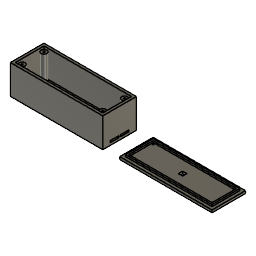
CajaSensorHumedad_v1 (Autodesk Fusion 360 design; units mm, degrees)
part number: 2026-06-22-22-06-37-882
Autodesk Fusion 360 part; units mm, degrees
sketch "Boceto1" plane through (0, 0, 0) normal (0, 0, 1) x (1, 0, 0)
sketch "Boceto2" plane through (0, 0, 0) normal (0, 0, 1) x (1, 0, 0)
sketch "Boceto3" plane through (0, 0, 0) normal (0, 0, 1) x (1, 0, 0)
  line L0 (0, 0) -> (110, 0)
  line L1 (110, 0) -> (110, 40)
  line L2 (110, 40) -> (0, 40)
  line L3 (0, 40) -> (0, 0)
sketch "Boceto4" plane through (0, 0, 0) normal (0, 0, 1) x (1, 0, 0)
  line L0 (0, 0) -> (110, 0)
  line L1 (110, 0) -> (110, 3)
  line L2 (110, 3) -> (0, 3)
  line L3 (0, 3) -> (0, 0)
sketch "Boceto5" plane through (0, 0, 0) normal (0, 0, 1) x (1, 0, 0)
  line L0 (0, 37) -> (110, 37)
  line L1 (110, 37) -> (110, 40)
  line L2 (110, 40) -> (0, 40)
  line L3 (0, 40) -> (0, 37)
sketch "Boceto6" plane through (0, 0, 0) normal (0, 0, 1) x (1, 0, 0)
  line L0 (0, 0) -> (3, 0)
  line L1 (3, 0) -> (3, 13)
  line L2 (3, 13) -> (0, 13)
  line L3 (0, 13) -> (0, 0)
sketch "Boceto7" plane through (0, 0, 0) normal (0, 0, 1) x (1, 0, 0)
  line L0 (0, 27) -> (3, 27)
  line L1 (3, 27) -> (3, 40)
  line L2 (3, 40) -> (0, 40)
  line L3 (0, 40) -> (0, 27)
sketch "Boceto8" plane through (0, 0, 0) normal (0, 0, 1) x (1, 0, 0)
  line L0 (0, 13) -> (3, 13)
  line L1 (3, 13) -> (3, 27)
  line L2 (3, 27) -> (0, 27)
  line L3 (0, 27) -> (0, 13)
sketch "Boceto9" plane through (0, 0, 0) normal (0, 0, 1) x (1, 0, 0)
  line L0 (107, 0) -> (110, 0)
  line L1 (110, 0) -> (110, 9)
  line L2 (110, 9) -> (107, 9)
  line L3 (107, 9) -> (107, 0)
sketch "Boceto10" plane through (0, 0, 0) normal (0, 0, 1) x (1, 0, 0)
  line L0 (107, 19) -> (110, 19)
  line L1 (110, 19) -> (110, 21)
  line L2 (110, 21) -> (107, 21)
  line L3 (107, 21) -> (107, 19)
sketch "Boceto11" plane through (0, 0, 0) normal (0, 0, 1) x (1, 0, 0)
  line L0 (107, 31) -> (110, 31)
  line L1 (110, 31) -> (110, 40)
  line L2 (110, 40) -> (107, 40)
  line L3 (107, 40) -> (107, 31)
sketch "Boceto12" plane through (0, 0, 0) normal (0, 0, 1) x (1, 0, 0)
  line L0 (107, 9) -> (110, 9)
  line L1 (110, 9) -> (110, 31)
  line L2 (110, 31) -> (107, 31)
  line L3 (107, 31) -> (107, 9)
sketch "Boceto13" plane through (0, 0, 0) normal (0, 0, 1) x (1, 0, 0)
  circle A0 centre (7, 7) radius 3.5
sketch "Boceto14" plane through (0, 0, 0) normal (0, 0, 1) x (1, 0, 0)
  circle A0 centre (7, 7) radius 1.1
sketch "Boceto15" plane through (0, 0, 0) normal (0, 0, 1) x (1, 0, 0)
  circle A0 centre (103, 7) radius 3.5
sketch "Boceto16" plane through (0, 0, 0) normal (0, 0, 1) x (1, 0, 0)
  circle A0 centre (103, 7) radius 1.1
sketch "Boceto17" plane through (0, 0, 0) normal (0, 0, 1) x (1, 0, 0)
  circle A0 centre (7, 33) radius 3.5
sketch "Boceto18" plane through (0, 0, 0) normal (0, 0, 1) x (1, 0, 0)
  circle A0 centre (7, 33) radius 1.1
sketch "Boceto19" plane through (0, 0, 0) normal (0, 0, 1) x (1, 0, 0)
  circle A0 centre (103, 33) radius 3.5
sketch "Boceto20" plane through (0, 0, 0) normal (0, 0, 1) x (1, 0, 0)
  circle A0 centre (103, 33) radius 1.1
sketch "Boceto21" plane through (0, 0, 0) normal (0, 0, 1) x (1, 0, 0)
  circle A0 centre (35, 12) radius 2.5
sketch "Boceto22" plane through (0, 0, 0) normal (0, 0, 1) x (1, 0, 0)
  circle A0 centre (35, 12) radius 1.1
sketch "Boceto23" plane through (0, 0, 0) normal (0, 0, 1) x (1, 0, 0)
  circle A0 centre (75, 12) radius 2.5
sketch "Boceto24" plane through (0, 0, 0) normal (0, 0, 1) x (1, 0, 0)
  circle A0 centre (75, 12) radius 1.1
sketch "Boceto25" plane through (0, 0, 0) normal (0, 0, 1) x (1, 0, 0)
  circle A0 centre (35, 28) radius 2.5
sketch "Boceto26" plane through (0, 0, 0) normal (0, 0, 1) x (1, 0, 0)
  circle A0 centre (35, 28) radius 1.1
sketch "Boceto27" plane through (0, 0, 0) normal (0, 0, 1) x (1, 0, 0)
  circle A0 centre (75, 28) radius 2.5
sketch "Boceto28" plane through (0, 0, 0) normal (0, 0, 1) x (1, 0, 0)
  circle A0 centre (75, 28) radius 1.1
sketch "Boceto29" plane through (0, 0, 0) normal (0, 0, 1) x (1, 0, 0)
  circle A0 centre (95, 20) radius 3
sketch "Boceto30" plane through (0, 0, 0) normal (0, 0, 1) x (1, 0, 0)
  circle A0 centre (95, 20) radius 1.6
sketch "Boceto31" plane through (0, 0, 0) normal (0, 0, 1) x (1, 0, 0)
  circle A0 centre (53, 20) radius 2.5
sketch "Boceto32" plane through (0, 0, 0) normal (0, 0, 1) x (1, 0, 0)
  circle A0 centre (53, 20) radius 1.1
sketch "Boceto33" plane through (0, 0, 0) normal (0, 0, 1) x (1, 0, 0)
  circle A0 centre (57, 20) radius 2.5
sketch "Boceto34" plane through (0, 0, 0) normal (0, 0, 1) x (1, 0, 0)
  circle A0 centre (57, 20) radius 1.1
sketch "Boceto35" plane through (0, 0, 0) normal (0, 0, 1) x (1, 0, 0)
  line L0 (130, 0) -> (240, 0)
  line L1 (240, 0) -> (240, 40)
  line L2 (240, 40) -> (130, 40)
  line L3 (130, 40) -> (130, 0)
sketch "Boceto36" plane through (0, 0, 0) normal (0, 0, 1) x (1, 0, 0)
  line L0 (133.5, 3.5) -> (236.5, 3.5)
  line L1 (236.5, 3.5) -> (236.5, 5.5)
  line L2 (236.5, 5.5) -> (133.5, 5.5)
  line L3 (133.5, 5.5) -> (133.5, 3.5)
sketch "Boceto37" plane through (0, 0, 0) normal (0, 0, 1) x (1, 0, 0)
  line L0 (133.5, 34.5) -> (236.5, 34.5)
  line L1 (236.5, 34.5) -> (236.5, 36.5)
  line L2 (236.5, 36.5) -> (133.5, 36.5)
  line L3 (133.5, 36.5) -> (133.5, 34.5)
sketch "Boceto38" plane through (0, 0, 0) normal (0, 0, 1) x (1, 0, 0)
  line L0 (133.5, 3.5) -> (135.5, 3.5)
  line L1 (135.5, 3.5) -> (135.5, 36.5)
  line L2 (135.5, 36.5) -> (133.5, 36.5)
  line L3 (133.5, 36.5) -> (133.5, 3.5)
sketch "Boceto39" plane through (0, 0, 0) normal (0, 0, 1) x (1, 0, 0)
  line L0 (234.5, 3.5) -> (236.5, 3.5)
  line L1 (236.5, 3.5) -> (236.5, 36.5)
  line L2 (236.5, 36.5) -> (234.5, 36.5)
  line L3 (234.5, 36.5) -> (234.5, 3.5)
sketch "Boceto40" plane through (0, 0, 0) normal (0, 0, 1) x (1, 0, 0)
  line L0 (182.5, 17.5) -> (187.5, 17.5)
  line L1 (187.5, 17.5) -> (187.5, 22.5)
  line L2 (187.5, 22.5) -> (182.5, 22.5)
  line L3 (182.5, 22.5) -> (182.5, 17.5)
sketch "Boceto41" plane through (0, 0, 0) normal (0, 0, 1) x (1, 0, 0)
  circle A0 centre (137, 7) radius 1.1
sketch "Boceto42" plane through (0, 0, 0) normal (0, 0, 1) x (1, 0, 0)
  circle A0 centre (233, 7) radius 1.1
sketch "Boceto43" plane through (0, 0, 0) normal (0, 0, 1) x (1, 0, 0)
  circle A0 centre (137, 33) radius 1.1
sketch "Boceto44" plane through (0, 0, 0) normal (0, 0, 1) x (1, 0, 0)
  circle A0 centre (233, 33) radius 1.1
sketch "Boceto45" plane through (0, 0, 0) normal (0, 0, 1) x (1, 0, 0)
  line L0 (0, 0) -> (110, 0)
  line L1 (110, 0) -> (110, 40)
  line L2 (110, 40) -> (0, 40)
  line L3 (0, 40) -> (0, 0)
sketch "Boceto46" plane through (0, 0, 0) normal (0, 0, 1) x (1, 0, 0)
  line L0 (0, 0) -> (110, 0)
  line L1 (110, 0) -> (110, 3)
  line L2 (110, 3) -> (0, 3)
  line L3 (0, 3) -> (0, 0)
sketch "Boceto47" plane through (0, 0, 0) normal (0, 0, 1) x (1, 0, 0)
  line L0 (0, 37) -> (110, 37)
  line L1 (110, 37) -> (110, 40)
  line L2 (110, 40) -> (0, 40)
  line L3 (0, 40) -> (0, 37)
sketch "Boceto48" plane through (0, 0, 0) normal (0, 0, 1) x (1, 0, 0)
  line L0 (0, 0) -> (3, 0)
  line L1 (3, 0) -> (3, 13)
  line L2 (3, 13) -> (0, 13)
  line L3 (0, 13) -> (0, 0)
sketch "Boceto49" plane through (0, 0, 0) normal (0, 0, 1) x (1, 0, 0)
  line L0 (0, 27) -> (3, 27)
  line L1 (3, 27) -> (3, 40)
  line L2 (3, 40) -> (0, 40)
  line L3 (0, 40) -> (0, 27)
sketch "Boceto50" plane through (0, 0, 0) normal (0, 0, 1) x (1, 0, 0)
  line L0 (0, 13) -> (3, 13)
  line L1 (3, 13) -> (3, 27)
  line L2 (3, 27) -> (0, 27)
  line L3 (0, 27) -> (0, 13)
sketch "Boceto51" plane through (0, 0, 0) normal (0, 0, 1) x (1, 0, 0)
  line L0 (107, 0) -> (110, 0)
  line L1 (110, 0) -> (110, 9)
  line L2 (110, 9) -> (107, 9)
  line L3 (107, 9) -> (107, 0)
sketch "Boceto52" plane through (0, 0, 0) normal (0, 0, 1) x (1, 0, 0)
  line L0 (107, 19) -> (110, 19)
  line L1 (110, 19) -> (110, 21)
  line L2 (110, 21) -> (107, 21)
  line L3 (107, 21) -> (107, 19)
sketch "Boceto53" plane through (0, 0, 0) normal (0, 0, 1) x (1, 0, 0)
  line L0 (107, 31) -> (110, 31)
  line L1 (110, 31) -> (110, 40)
  line L2 (110, 40) -> (107, 40)
  line L3 (107, 40) -> (107, 31)
sketch "Boceto54" plane through (0, 0, 0) normal (0, 0, 1) x (1, 0, 0)
  line L0 (107, 9) -> (110, 9)
  line L1 (110, 9) -> (110, 31)
  line L2 (110, 31) -> (107, 31)
  line L3 (107, 31) -> (107, 9)
sketch "Boceto55" plane through (0, 0, 0) normal (0, 0, 1) x (1, 0, 0)
  circle A0 centre (7, 7) radius 3.5
sketch "Boceto56" plane through (0, 0, 0) normal (0, 0, 1) x (1, 0, 0)
  circle A0 centre (7, 7) radius 1.1
sketch "Boceto57" plane through (0, 0, 0) normal (0, 0, 1) x (1, 0, 0)
  circle A0 centre (103, 7) radius 3.5
sketch "Boceto58" plane through (0, 0, 0) normal (0, 0, 1) x (1, 0, 0)
  circle A0 centre (103, 7) radius 1.1
sketch "Boceto59" plane through (0, 0, 0) normal (0, 0, 1) x (1, 0, 0)
  circle A0 centre (7, 33) radius 3.5
sketch "Boceto60" plane through (0, 0, 0) normal (0, 0, 1) x (1, 0, 0)
  circle A0 centre (7, 33) radius 1.1
sketch "Boceto61" plane through (0, 0, 0) normal (0, 0, 1) x (1, 0, 0)
  circle A0 centre (103, 33) radius 3.5
sketch "Boceto62" plane through (0, 0, 0) normal (0, 0, 1) x (1, 0, 0)
  circle A0 centre (103, 33) radius 1.1
sketch "Boceto63" plane through (0, 0, 0) normal (0, 0, 1) x (1, 0, 0)
  line L0 (130, 0) -> (240, 0)
  line L1 (240, 0) -> (240, 40)
  line L2 (240, 40) -> (130, 40)
  line L3 (130, 40) -> (130, 0)
sketch "Boceto64" plane through (0, 0, 0) normal (0, 0, 1) x (1, 0, 0)
  line L0 (133.5, 3.5) -> (236.5, 3.5)
  line L1 (236.5, 3.5) -> (236.5, 5.5)
  line L2 (236.5, 5.5) -> (133.5, 5.5)
  line L3 (133.5, 5.5) -> (133.5, 3.5)
sketch "Boceto65" plane through (0, 0, 0) normal (0, 0, 1) x (1, 0, 0)
  line L0 (133.5, 34.5) -> (236.5, 34.5)
  line L1 (236.5, 34.5) -> (236.5, 36.5)
  line L2 (236.5, 36.5) -> (133.5, 36.5)
  line L3 (133.5, 36.5) -> (133.5, 34.5)
sketch "Boceto66" plane through (0, 0, 0) normal (0, 0, 1) x (1, 0, 0)
  line L0 (133.5, 3.5) -> (135.5, 3.5)
  line L1 (135.5, 3.5) -> (135.5, 36.5)
  line L2 (135.5, 36.5) -> (133.5, 36.5)
  line L3 (133.5, 36.5) -> (133.5, 3.5)
sketch "Boceto67" plane through (0, 0, 0) normal (0, 0, 1) x (1, 0, 0)
  line L0 (234.5, 3.5) -> (236.5, 3.5)
  line L1 (236.5, 3.5) -> (236.5, 36.5)
  line L2 (236.5, 36.5) -> (234.5, 36.5)
  line L3 (234.5, 36.5) -> (234.5, 3.5)
sketch "Boceto68" plane through (0, 0, 0) normal (0, 0, 1) x (1, 0, 0)
  line L0 (182.5, 17.5) -> (187.5, 17.5)
  line L1 (187.5, 17.5) -> (187.5, 22.5)
  line L2 (187.5, 22.5) -> (182.5, 22.5)
  line L3 (182.5, 22.5) -> (182.5, 17.5)
sketch "Boceto69" plane through (0, 0, 0) normal (0, 0, 1) x (1, 0, 0)
  circle A0 centre (137, 7) radius 1.1
sketch "Boceto70" plane through (0, 0, 0) normal (0, 0, 1) x (1, 0, 0)
  circle A0 centre (233, 7) radius 1.1
sketch "Boceto71" plane through (0, 0, 0) normal (0, 0, 1) x (1, 0, 0)
  circle A0 centre (137, 33) radius 1.1
sketch "Boceto72" plane through (0, 0, 0) normal (0, 0, 1) x (1, 0, 0)
  circle A0 centre (233, 33) radius 1.1
sketch "Boceto73" plane through (0, 0, 0) normal (0, 0, 1) x (1, 0, 0)
  line L0 (0, 0) -> (110, 0)
  line L1 (110, 0) -> (110, 40)
  line L2 (110, 40) -> (0, 40)
  line L3 (0, 40) -> (0, 0)
extrude "Extruir71" add sketch "Boceto73" along normal blind 3 makes body 1
sketch "Boceto74" plane through (0, 0, 0) normal (0, 0, 1) x (1, 0, 0)
  line L0 (0, 0) -> (110, 0)
  line L1 (110, 0) -> (110, 3)
  line L2 (110, 3) -> (0, 3)
  line L3 (0, 3) -> (0, 0)
extrude "Extruir72" add sketch "Boceto74" along normal blind 32 separate body makes body 2
move_body "Desplazar42" bodies 2 to x (1, 0, 0) y (0, 1, 0) z (0, 0, 1) at (0, 0, 3)
sketch "Boceto75" plane through (0, 0, 0) normal (0, 0, 1) x (1, 0, 0)
  line L0 (0, 37) -> (110, 37)
  line L1 (110, 37) -> (110, 40)
  line L2 (110, 40) -> (0, 40)
  line L3 (0, 40) -> (0, 37)
extrude "Extruir73" add sketch "Boceto75" along normal blind 32 separate body makes body 3
move_body "Desplazar43" bodies 3 to x (1, 0, 0) y (0, 1, 0) z (0, 0, 1) at (0, 0, 3)
sketch "Boceto76" plane through (0, 0, 0) normal (0, 0, 1) x (1, 0, 0)
  line L0 (0, 0) -> (3, 0)
  line L1 (3, 0) -> (3, 13)
  line L2 (3, 13) -> (0, 13)
  line L3 (0, 13) -> (0, 0)
extrude "Extruir74" add sketch "Boceto76" along normal blind 32 separate body makes body 4
move_body "Desplazar44" bodies 4 to x (1, 0, 0) y (0, 1, 0) z (0, 0, 1) at (0, 0, 3)
sketch "Boceto77" plane through (0, 0, 0) normal (0, 0, 1) x (1, 0, 0)
  line L0 (0, 27) -> (3, 27)
  line L1 (3, 27) -> (3, 40)
  line L2 (3, 40) -> (0, 40)
  line L3 (0, 40) -> (0, 27)
extrude "Extruir75" add sketch "Boceto77" along normal blind 32 separate body makes body 5
move_body "Desplazar45" bodies 5 to x (1, 0, 0) y (0, 1, 0) z (0, 0, 1) at (0, 0, 3)
sketch "Boceto78" plane through (0, 0, 0) normal (0, 0, 1) x (1, 0, 0)
  line L0 (0, 13) -> (3, 13)
  line L1 (3, 13) -> (3, 27)
  line L2 (3, 27) -> (0, 27)
  line L3 (0, 27) -> (0, 13)
extrude "Extruir76" add sketch "Boceto78" along normal blind 24 separate body makes body 6
move_body "Desplazar46" bodies 6 to x (1, 0, 0) y (0, 1, 0) z (0, 0, 1) at (0, 0, 11)
sketch "Boceto79" plane through (0, 0, 0) normal (0, 0, 1) x (1, 0, 0)
  line L0 (107, 0) -> (110, 0)
  line L1 (110, 0) -> (110, 9)
  line L2 (110, 9) -> (107, 9)
  line L3 (107, 9) -> (107, 0)
extrude "Extruir77" add sketch "Boceto79" along normal blind 32 separate body makes body 7
move_body "Desplazar47" bodies 7 to x (1, 0, 0) y (0, 1, 0) z (0, 0, 1) at (0, 0, 3)
sketch "Boceto80" plane through (0, 0, 0) normal (0, 0, 1) x (1, 0, 0)
  line L0 (107, 19) -> (110, 19)
  line L1 (110, 19) -> (110, 21)
  line L2 (110, 21) -> (107, 21)
  line L3 (107, 21) -> (107, 19)
extrude "Extruir78" add sketch "Boceto80" along normal blind 2 separate body makes body 8
move_body "Desplazar48" bodies 8 to x (1, 0, 0) y (0, 1, 0) z (0, 0, 1) at (0, 0, 3)
sketch "Boceto81" plane through (0, 0, 0) normal (0, 0, 1) x (1, 0, 0)
  line L0 (107, 31) -> (110, 31)
  line L1 (110, 31) -> (110, 40)
  line L2 (110, 40) -> (107, 40)
  line L3 (107, 40) -> (107, 31)
extrude "Extruir79" add sketch "Boceto81" along normal blind 32 separate body makes body 9
move_body "Desplazar49" bodies 9 to x (1, 0, 0) y (0, 1, 0) z (0, 0, 1) at (0, 0, 3)
sketch "Boceto82" plane through (0, 0, 0) normal (0, 0, 1) x (1, 0, 0)
  line L0 (107, 9) -> (110, 9)
  line L1 (110, 9) -> (110, 31)
  line L2 (110, 31) -> (107, 31)
  line L3 (107, 31) -> (107, 9)
extrude "Extruir80" add sketch "Boceto82" along normal blind 30 separate body makes body 10
move_body "Desplazar50" bodies 10 to x (1, 0, 0) y (0, 1, 0) z (0, 0, 1) at (0, 0, 5)
sketch "Boceto83" plane through (0, 0, 0) normal (0, 0, 1) x (1, 0, 0)
  circle A0 centre (7, 7) radius 3.5
extrude "Extruir81" add sketch "Boceto83" along normal blind 30 separate body makes body 11
move_body "Desplazar51" bodies 11 to x (1, 0, 0) y (0, 1, 0) z (0, 0, 1) at (0, 0, 3)
sketch "Boceto84" plane through (0, 0, 0) normal (0, 0, 1) x (1, 0, 0)
  circle A0 centre (7, 7) radius 1.1
extrude "Extruir82" cut sketch "Boceto84" along normal blind 37 bodies 1 11
sketch "Boceto85" plane through (0, 0, 0) normal (0, 0, 1) x (1, 0, 0)
  circle A0 centre (103, 7) radius 3.5
extrude "Extruir83" add sketch "Boceto85" along normal blind 30 separate body makes body 12
move_body "Desplazar52" bodies 12 to x (1, 0, 0) y (0, 1, 0) z (0, 0, 1) at (0, 0, 3)
sketch "Boceto86" plane through (0, 0, 0) normal (0, 0, 1) x (1, 0, 0)
  circle A0 centre (103, 7) radius 1.1
extrude "Extruir84" cut sketch "Boceto86" along normal blind 37 bodies 1 12
sketch "Boceto87" plane through (0, 0, 0) normal (0, 0, 1) x (1, 0, 0)
  circle A0 centre (7, 33) radius 3.5
extrude "Extruir85" add sketch "Boceto87" along normal blind 30 separate body makes body 13
move_body "Desplazar53" bodies 13 to x (1, 0, 0) y (0, 1, 0) z (0, 0, 1) at (0, 0, 3)
sketch "Boceto88" plane through (0, 0, 0) normal (0, 0, 1) x (1, 0, 0)
  circle A0 centre (7, 33) radius 1.1
extrude "Extruir86" cut sketch "Boceto88" along normal blind 37 bodies 1 13
sketch "Boceto89" plane through (0, 0, 0) normal (0, 0, 1) x (1, 0, 0)
  circle A0 centre (103, 33) radius 3.5
extrude "Extruir87" add sketch "Boceto89" along normal blind 30 separate body makes body 14
move_body "Desplazar54" bodies 14 to x (1, 0, 0) y (0, 1, 0) z (0, 0, 1) at (0, 0, 3)
sketch "Boceto90" plane through (0, 0, 0) normal (0, 0, 1) x (1, 0, 0)
  circle A0 centre (103, 33) radius 1.1
extrude "Extruir88" cut sketch "Boceto90" along normal blind 37 bodies 1 14
sketch "Boceto91" plane through (0, 0, 0) normal (0, 0, 1) x (1, 0, 0)
  line L0 (130, 0) -> (240, 0)
  line L1 (240, 0) -> (240, 40)
  line L2 (240, 40) -> (130, 40)
  line L3 (130, 40) -> (130, 0)
extrude "Extruir89" add sketch "Boceto91" along normal blind 3 separate body makes body 15
sketch "Boceto92" plane through (0, 0, 0) normal (0, 0, 1) x (1, 0, 0)
  line L0 (133.5, 3.5) -> (236.5, 3.5)
  line L1 (236.5, 3.5) -> (236.5, 5.5)
  line L2 (236.5, 5.5) -> (133.5, 5.5)
  line L3 (133.5, 5.5) -> (133.5, 3.5)
extrude "Extruir90" add sketch "Boceto92" along normal blind 2 separate body makes body 16
move_body "Desplazar55" bodies 16 to x (1, 0, 0) y (0, 1, 0) z (0, 0, 1) at (0, 0, 3)
sketch "Boceto93" plane through (0, 0, 0) normal (0, 0, 1) x (1, 0, 0)
  line L0 (133.5, 34.5) -> (236.5, 34.5)
  line L1 (236.5, 34.5) -> (236.5, 36.5)
  line L2 (236.5, 36.5) -> (133.5, 36.5)
  line L3 (133.5, 36.5) -> (133.5, 34.5)
extrude "Extruir91" add sketch "Boceto93" along normal blind 2 separate body makes body 17
move_body "Desplazar56" bodies 17 to x (1, 0, 0) y (0, 1, 0) z (0, 0, 1) at (0, 0, 3)
sketch "Boceto94" plane through (0, 0, 0) normal (0, 0, 1) x (1, 0, 0)
  line L0 (133.5, 3.5) -> (135.5, 3.5)
  line L1 (135.5, 3.5) -> (135.5, 36.5)
  line L2 (135.5, 36.5) -> (133.5, 36.5)
  line L3 (133.5, 36.5) -> (133.5, 3.5)
extrude "Extruir92" add sketch "Boceto94" along normal blind 2 separate body makes body 18
move_body "Desplazar57" bodies 18 to x (1, 0, 0) y (0, 1, 0) z (0, 0, 1) at (0, 0, 3)
sketch "Boceto95" plane through (0, 0, 0) normal (0, 0, 1) x (1, 0, 0)
  line L0 (234.5, 3.5) -> (236.5, 3.5)
  line L1 (236.5, 3.5) -> (236.5, 36.5)
  line L2 (236.5, 36.5) -> (234.5, 36.5)
  line L3 (234.5, 36.5) -> (234.5, 3.5)
extrude "Extruir93" add sketch "Boceto95" along normal blind 2 separate body makes body 19
move_body "Desplazar58" bodies 19 to x (1, 0, 0) y (0, 1, 0) z (0, 0, 1) at (0, 0, 3)
sketch "Boceto96" plane through (0, 0, 0) normal (0, 0, 1) x (1, 0, 0)
  line L0 (182.5, 17.5) -> (187.5, 17.5)
  line L1 (187.5, 17.5) -> (187.5, 22.5)
  line L2 (187.5, 22.5) -> (182.5, 22.5)
  line L3 (182.5, 22.5) -> (182.5, 17.5)
extrude "Extruir94" cut sketch "Boceto96" along normal blind 5 bodies 15
sketch "Boceto97" plane through (0, 0, 0) normal (0, 0, 1) x (1, 0, 0)
  circle A0 centre (137, 7) radius 1.1
extrude "Extruir95" cut sketch "Boceto97" along normal blind 5 bodies 15
sketch "Boceto98" plane through (0, 0, 0) normal (0, 0, 1) x (1, 0, 0)
  circle A0 centre (233, 7) radius 1.1
extrude "Extruir96" cut sketch "Boceto98" along normal blind 5 bodies 15
sketch "Boceto99" plane through (0, 0, 0) normal (0, 0, 1) x (1, 0, 0)
  circle A0 centre (137, 33) radius 1.1
extrude "Extruir97" cut sketch "Boceto99" along normal blind 5 bodies 15
sketch "Boceto100" plane through (0, 0, 0) normal (0, 0, 1) x (1, 0, 0)
  circle A0 centre (233, 33) radius 1.1
extrude "Extruir98" cut sketch "Boceto100" along normal blind 5 bodies 15
combine "Combinar1" operation add target body 1 tool bodies 2 3 4 5 6 7 8 9 10 11 12 13 14
combine "Combinar2" operation add target body 15 tool bodies 16 17 18 19
named bodies: "Piso liso caja", "Pared lateral 1", "Pared lateral 2", "Pared USB izquierda", "Pared USB derecha", "Puente superior USB", "Pared sensor izquierda", "Separador sensor central", "Pared sensor derecha", "Puente superior sensor", "Poste tornillo tapa", "Poste tornillo tapa (1)", "Poste tornillo tapa (2)", "Poste tornillo tapa (3)", "Tapa superior", "Labio tapa inferior", "Labio tapa superior", "Labio tapa izquierdo", "Labio tapa derecho"
